Encoder Bracket_v1 (Autodesk Fusion 360 design; units mm, degrees)
Autodesk Fusion 360 part; units mm, degrees
note: some values were not read from the file. Set by a fixed rule: which sketch regions a step uses.
sketch "Sketch1" plane through (0, 0, 0) normal (0, 0, 1) x (1, 0, 0)
  line L0 (5.5, 9) -> (-5.5, 9) construction
  line L1 (-5.5, 9) -> (-5.5, -9) construction
  line L2 (-5.5, -9) -> (5.5, -9) construction
  line L3 (5.5, -9) -> (5.5, 9) construction
  line L4 (5.5, 9) -> (-5.5, -9) construction
  line L5 (-5.5, 9) -> (5.5, -9) construction
  line L6 (7, -10.5) -> (-7, -10.5)
  line L7 (-7, -10.5) -> (-7, 10.5)
  line L8 (-7, 10.5) -> (7, 10.5)
  line L9 (7, 10.5) -> (7, -10.5)
  line L10 (7, -10.5) -> (-7, 10.5) construction
  line L11 (-7, -10.5) -> (7, 10.5) construction
  line L12 (4.5, -8) -> (-4.5, -8)
  line L13 (-4.5, -8) -> (-4.5, 8)
  line L14 (-4.5, 8) -> (4.5, 8)
  line L15 (4.5, 8) -> (4.5, -8)
  line L16 (4.5, -8) -> (-4.5, 8) construction
  line L17 (-4.5, -8) -> (4.5, 8) construction
  circle A0 centre (-5.5, 9) radius 1.05
  circle A1 centre (5.5, 9) radius 1.05
  circle A2 centre (5.5, -9) radius 1.05
  circle A3 centre (-5.5, -9) radius 1.05
  line L18 (-4.5, 8) -> (4.5, 8)
  line L19 (4.5, 8) -> (4.5, -10.5)
  line L20 (4.5, -10.5) -> (-4.5, -10.5)
  line L21 (-4.5, -10.5) -> (-4.5, 8)
  line L22 (4.5, 8) -> (-7, 8)
  line L23 (-7, 8) -> (-7, -8)
  line L24 (-7, -8) -> (4.5, -8)
  line L25 (4.5, -8) -> (4.5, 8)
  dimension "d1" = 11
  dimension "d2" = 18
  dimension "d3" = 14
  dimension "d4" = 21
  dimension "d5" = 9
  dimension "d6" = 16
  dimension "d7" = 2.1
  dimension "d8" = 2.1
  dimension "d9" = 2.1
  dimension "d10" = 2.1
  dimension "d11" = 9
  constraint horizontal L0
  constraint perpendicular L0 L1
  constraint parallel L0 L2
  constraint parallel L1 L3
  constraint coincident L4 origin
  constraint coincident L5 origin
  constraint horizontal L6
  constraint perpendicular L6 L7
  constraint parallel L6 L8
  constraint parallel L7 L9
  constraint coincident L10 origin
  constraint coincident L11 origin
  constraint horizontal L12
  constraint perpendicular L12 L13
  constraint parallel L12 L14
  constraint parallel L13 L15
  constraint coincident L16 origin
  constraint coincident L17 origin
  constraint coincident L0.end L1.start
  constraint coincident L0.start L3.end
  constraint coincident L2.end L3.start
  constraint coincident L1.end L2.start
  constraint horizontal L18
  constraint vertical L19
  constraint horizontal L20
  constraint vertical L21
  constraint horizontal L22
  constraint vertical L23
  constraint horizontal L24
  constraint vertical L25
  constraint coincident L7 L23.end
  measures "d1" distance of L1.end L2.end
  measures "d2" distance of L0.end L1.end
  measures "d3" distance of L7.end L8.end
  measures "d4" distance of L6.end L7.end
  measures "d5" distance of L13.end L14.end
  measures "d6" distance of L12.end L13.end
  measures "d7" diameter of A0
  measures "d8" diameter of A1
  measures "d9" diameter of A2
  measures "d10" diameter of A3
  measures "d11" distance of L13.end L14.end
extrude "Extrude1" add sketch "Sketch1" along normal blind 2 contours L6 L7 L8 L9 L14 L15 A0 A2 L18 L19 L22 L25 | L6 L12 A2 A3 L19 L20 L21 L24 | L6 L7 A3 L21 L24 | A3 L21 L24 picked at (-4.6728, -8.1728)
